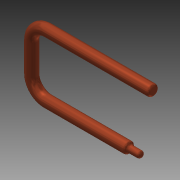
# Autodesk Inventor part: Copper_tube
Saved by Autodesk Inventor 2015 (Build 190159000, 159)
## iProperties
Created: 2015-08-22
Part Number: Copper_tube
Material: Copper
Document SubType Name: Modeling
Designer: Kyle
Density: 8.94 g/cm^3
Appearance: Copper - Satin
Author: Kyle
Autodesk Inventor part; units mm, degrees
ref_plane "YZ Plane" through (0, 0, 0) normal (1, 0, 0) x (0, 1, 0)
ref_plane "XZ Plane" through (0, 0, 0) normal (0, 1, 0) x (-1, 0, 0)
ref_plane "XY Plane" through (0, 0, 0) normal (0, 0, 1) x (1, 0, 0)
sketch "Sketch1" plane through (0, 0, 0) normal (0, 0, 1) x (1, 0, 0)
  line L0 (0, 3.175) -> (0, -3.175)
  line L1 (0, -3.175) -> (-61.595, -3.175)
  line L2 (0, 3.175) -> (-61.595, 3.175)
  line L3 (-61.595, -33.3502) -> (-14.4526, -33.3502)
  line L4 (-61.595, -39.7002) -> (-14.4526, -39.7002)
  line L5 (-14.4526, -39.7002) -> (-14.4526, -38.4302)
  line L6 (-14.4526, -33.3502) -> (-14.4526, -34.6202)
  line L7 (-69.215, -13.1699) -> (-69.215, -23.3299)
  line L8 (-75.565, -13.1699) -> (-75.565, -23.3299)
  line L9 (-69.215, -13.1699) -> (-69.215, -3.175)
  line L10 (-69.215, -3.175) -> (-61.595, -3.175)
  line L11 (-61.595, 3.175) -> (-75.565, 3.175)
  line L12 (-75.565, 3.175) -> (-75.565, -13.1699)
  line L13 (-75.565, -23.3299) -> (-75.565, -39.7002)
  line L14 (-75.565, -39.7002) -> (-61.595, -39.7002)
  line L15 (-61.595, -33.3502) -> (-69.215, -33.3502)
  line L16 (-69.215, -33.3502) -> (-69.215, -23.3299)
  line L17 (-14.4526, -34.6202) -> (-14.4526, -38.4302)
  point P0 (0, 0)
  point P1 (0, 0)
  point P2 (-61.595, 0)
  point P3 (-72.39, -18.2499)
  point P4 (-72.39, -13.1699)
  point P5 (-72.39, -23.3299)
  point P6 (-14.4526, -36.5252)
  dimension "d0" = 61.595
  dimension "d1" = 18.2499
  dimension "d2" = 10.795
  dimension "d3" = 5.08
  dimension "d4" = 5.08
  dimension "d8" = 3.175
  dimension "d9" = 3.175
  dimension "d10" = 3.175
  dimension "d11" = 3.175
  dimension "d12" = 1.905
  dimension "d13" = 1.905
  dimension "d14" = 3.175
  dimension "d15" = 3.175
  dimension "d35" = 36.5252
  constraints: 36 end point, 7 vertical, 5 horizontal, 4 perpendicular, 2 point on line, 1 coincident, 1 parallel
  measures "d0" distance of point (-61.595, 0) point (0, 0)
  measures "d1" vertical distance of point (-72.39, -18.25) point (-61.595, 0)
  measures "d2" horizontal distance of point (-72.39, -18.25) point (-61.595, 0)
  measures "d3" distance of point (-72.39, -18.25) point (-72.39, -13.17)
  measures "d4" distance of point (-72.39, -23.33) point (-72.39, -18.25)
  measures "d8" distance of point (0, 0) L0.start
  measures "d9" distance of point (0, 0) L0.end
  measures "d10" distance from line of point (-14.453, -36.525) L3
  measures "d11" distance from line of point (-14.453, -36.525) L4
  measures "d12" distance of L5.end point (-14.453, -36.525)
  measures "d13" distance of L6.end point (-14.453, -36.525)
  measures "d14" distance from line of point (-72.39, -13.17) L7
  measures "d15" distance from line of L8 point (-72.39, -13.17)
  measures "d35" vertical distance of point (0, 0) point (-14.453, -36.525)
extrude "Extrusion1" add sketch "Sketch1" along normal blind 6.35
sketch "Sketch2" plane through (-14.4526, -39.7002, 0) normal (1, 0, 0) x (0, 0, -1)
  line L0 (-5.08, 1.27) -> (-1.27, 1.27)
  line L1 (-1.27, 1.27) -> (-1.27, 5.08)
  line L2 (-1.27, 5.08) -> (-5.08, 5.08)
  line L3 (-5.08, 5.08) -> (-5.08, 1.27)
  line L4 (0, 6.35) -> (0, 0) projected
  line L5 (-6.35, 0) -> (-6.35, 6.35) projected
  line L6 (0, 0) -> (-6.35, 0) projected
  line L7 (0, 6.35) -> (-6.35, 6.35) projected
  point P0 (0, 39.7002)
  dimension "d18" = 1.27
  dimension "d19" = 1.27
  dimension "d20" = 1.27
  dimension "d21" = 1.27
  constraints: 8 end point, 2 parallel, 1 horizontal, 1 perpendicular
  measures "d18" distance between parallel lines of L4 L1
  measures "d19" distance between parallel lines of L5 L3
  measures "d20" distance between parallel lines of L6 L0
  measures "d21" distance between parallel lines of L7 L2
extrude "Extrusion2" add sketch "Sketch2" along normal blind 7.4422 contours L3 L2 L1 L0
fillet "Fillet3" radius 1.905 4 edges at (-10.7315, -34.6202, 5.08) (-10.7315, -34.6202, 1.27) (-10.7315, -38.4302, 1.27) (-10.7315, -38.4302, 5.08)
fillet "Fillet4" radius 1.27 8 edges at (-7.0104, -34.6202, 3.175) (-7.0104, -35.1781, 1.8279) (-7.0104, -35.1781, 4.5221) (-7.0104, -36.5252, 1.27) (-7.0104, -36.5252, 5.08) (-7.0104, -37.8723, 1.8279) (-7.0104, -37.8723, 4.5221) (-7.0104, -38.4302, 3.175)
fillet "Fillet5" radius 1.27 8 edges at (-14.4526, -34.6202, 3.175) (-14.4526, -35.1781, 1.8279) (-14.4526, -35.1781, 4.5221) (-14.4526, -36.5252, 1.27) (-14.4526, -36.5252, 5.08) (-14.4526, -37.8723, 1.8279) (-14.4526, -37.8723, 4.5221) (-14.4526, -38.4302, 3.175)
fillet "Fillet7" radius 12.7 1 edges at (-75.565, 3.175, 3.175)
fillet "Fillet8" radius 12.7 1 edges at (-75.565, -39.7002, 3.175)
fillet "Fillet9" radius 6.35 2 edges at (-69.215, -33.3502, 3.175) (-69.215, -3.175, 3.175)
fillet "Fillet10" radius 3.175 20 edges at (-71.8453, -0.5447, 6.35) (-75.565, -18.2626, 6.35) (-71.8453, -35.9805, 6.35) (-38.6588, -39.7002, 6.35) (-31.4325, 3.175, 6.35) (-71.8453, -0.5447, 0) (-75.565, -18.2626, 0) (-71.8453, -35.9805, 0) (-38.6588, -39.7002, 0) (-31.4325, 3.175, 0) (-67.3551, -5.0349, 6.35) (-69.215, -18.2626, 6.35) (-67.3551, -31.4903, 6.35) (-38.6588, -33.3502, 6.35) (-31.4325, -3.175, 6.35) (-67.3551, -31.4903, 0) (-69.215, -18.2626, 0) (-67.3551, -5.0349, 0) (-31.4325, -3.175, 0) (-38.6588, -33.3502, 0)
fillet "Fillet11" radius 1.27 24 edges at (0, 0, 6.35) (0, 2.2451, 5.4201) (0, -2.2451, 5.4201) (0, 3.175, 3.175) (0, 2.2451, 0.9299) (0, 0, 0) (0, -2.2451, 0.9299) (0, -3.175, 3.175) (-14.4526, -36.5252, 6.35) (-14.4526, -33.3502, 3.175) (-14.4526, -34.2801, 0.9299) (-14.4526, -34.2801, 5.4201) (-14.4526, -36.5252, 0) (-14.4526, -38.7703, 0.9299) (-14.4526, -38.7703, 5.4201) (-14.4526, -39.7002, 3.175) (-14.4526, -33.3503, 3.175) (-14.4526, -34.2802, 0.93) (-14.4526, -34.2802, 5.42) (-14.4526, -36.5252, 0.0001) (-14.4526, -36.5252, 6.3499) (-14.4526, -38.7702, 0.93) (-14.4526, -38.7702, 5.42) (-14.4526, -39.7001, 3.175)
body "Solid1"
